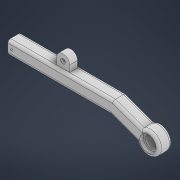
# Autodesk Inventor part: Fahrwerk_rocker_hinten
Saved by Autodesk Inventor 2021 (Build 250183000, 183)
## iProperties
Created: 2020-12-28
Part Number: Fahrwerk_rocker_hinten
Material: Generisch
Document SubType Name: Modeling
Designer: laure
Density: 1 g/cm^3
Appearance: Vorgabe
Author: laure
Autodesk Inventor part; units mm, degrees
ref_plane "YZ Plane" through (0, 0, 0) normal (1, 0, 0) x (0, 1, 0)
ref_plane "XZ Plane" through (0, 0, 0) normal (0, 1, 0) x (-1, 0, 0)
ref_plane "XY Plane" through (0, 0, 0) normal (0, 0, 1) x (1, 0, 0)
sketch "Skizze1" plane through (0, 0, 0) normal (0, 0, 1) x (1, 0, 0)
  line L0 (-110, 10) -> (50, 10)
  line L1 (46.4735, -10) -> (-110, -10)
  line L2 (-153.2763, 0) -> (149.6579, 0) projected
  line L3 (99.5412, -29.3151) -> (46.4735, -10)
  line L4 (50, 10) -> (106.3816, -10.5212)
  line L5 (106.3816, -10.5212) -> (99.5412, -29.3151)
  line L6 (0, -40.3885) -> (0, 37.1255) projected
  line L7 (-110, 10) -> (-110, -10)
  point P0 (0, 0)
  dimension "d5" = 20
  dimension "d56" = 0
  dimension "d57" = 0
  dimension "d58" = 60
  dimension "d138" = 160
  dimension "d140" = 20
  dimension "d141" = 10
  dimension "d142" = 110
  dimension "d143" = 50
  dimension "d144" = 10
  constraints: 12 end point, 2 parallel, 2 perpendicular, 1 horizontal, 1 other
  measures "d5" distance between parallel lines of L4 L3
  measures "d56" distance from line of L0 L4.start
  measures "d57" distance of L0.end L4.start
  measures "d58" distance from line of L4.start L5
  measures "d138" distance from line of L7 L0.end
  measures "d140" angle of L6 L5
  measures "d141" distance between parallel lines of L2 L0
  measures "d142" distance between parallel lines of L6 L7
  measures "d143" distance from line of point (50, 10) L6
  measures "d144" distance from line of point (50, 10) L2
sketch "Skizze4" plane through (0, 0, 0) normal (0, 0, 1) x (1, 0, 0)
  line L0 (-40, 10) -> (-20, 10)
  line L1 (-20, 10) -> (-20, 20)
  line L2 (-30, 30) -> (-30, 30)
  line L3 (-40, 20) -> (-40, 10)
  arc A0 (-30, 30) -> (-40, 20) centre (-30, 20) ccw
  arc A1 (-20, 20) -> (-30, 30) centre (-30, 20) ccw
  line L4 (-50.4853, 0) -> (8.4142, 0) projected
  line L5 (0, -6.4142) -> (0, 38.4853) projected
  line L6 (-35, 25) -> (-25, 25)
  line L7 (-25, 25) -> (-25, 15)
  line L8 (-25, 15) -> (-35, 15)
  line L9 (-35, 15) -> (-35, 25)
  line L10 (-35, 25) -> (-25, 15) construction
  line L11 (-25, 25) -> (-35, 15) construction
  point P0 (0, 0)
  point P1 (-30, 30)
  dimension "d74" = 20
  dimension "d75" = 20
  dimension "d78" = 10
  dimension "d116" = 10
  dimension "d160" = 10
  dimension "d161" = 10
  dimension "d162" = 20
  dimension "d167" = 10
  constraints: 20 end point, 4 parallel, 4 point on circle, 4 tangent, 2 centre point, 2 horizontal, 2 midpoint, 2 perpendicular, 1 concentric
  measures "d74" distance between parallel lines of L1 L3
  measures "d75" distance between parallel lines of L0 L2
  measures "d78" radius of A0
  measures "d116" distance between parallel lines of L0 L4
  measures "d160" distance of L7.end L8.end
  measures "d161" distance of L6.end L7.end
  measures "d162" distance between parallel lines of L5 L1
  measures "d167" distance from line of L0 A1.centre
extrude "Extrusion1" add sketch "Skizze1" against normal mid plane 20
sketch "Skizze13" plane through (0, 0, -10) normal (0, 0, -1) x (-1, 0, 0)
  line L0 (-106.3816, -10.5212) -> (-99.5412, -29.3151) projected
  circle A0 centre (-102.9614, -19.9181) radius 12.15
  circle A1 centre (-102.9614, -19.9181) radius 17
  point P0 (0, 0)
  point P1 (-105.5778, -12.7295)
  point P2 (-100.3449, -27.1068)
  dimension "d148" = 24.3
  dimension "d149" = 34
  constraints: 2 centre point, 1 coincident, 1 midpoint
  measures "d148" diameter of A0
  measures "d149" diameter of A1
extrude "Extrusion13" add sketch "Skizze13" against normal blind 20
extrude "Extrusion14" cut sketch "Skizze13" against normal up to surface (20 mm away) contours A0
shell "Wandung2" thickness 2.6 removed faces 1 at (-110, -3.3333, -3.3333)
extrude "Extrusion11" add sketch "Skizze4" against normal mid plane 12 contours L3 A0 A1 L1 L0 | L6 L7 L8 L9
sketch "Skizze12" plane through (0, 0, 10) normal (0, 0, 1) x (1, 0, 0)
  circle A0 centre (-104, 0) radius 1.6
  line L0 (-110, 6) -> (49.2947, 6) projected
  line L1 (-110, 10) -> (-110, -10) projected
  line L2 (50, 10) -> (-110, 10) projected
  point P0 (0, 0)
  point P1 (-110, -6)
  dimension "d133" = 3.2
  dimension "d135" = 6
  dimension "d147" = 10
  constraints: 1 centre point
  measures "d133" diameter of A0
  measures "d135" distance from line of L1 A0.centre
  measures "d147" distance from line of A0.centre L2
extrude "Extrusion12" cut sketch "Skizze12" against normal up to surface (20 mm away)
sketch "Skizze14" plane through (0, 0, 0) normal (0, 0, 1) x (1, 0, 0)
  circle A0 centre (102.9614, -19.9181) radius 12.15 projected
  circle A1 centre (102.9614, -19.9181) radius 9
  point P0 (0, 0)
  dimension "d157" = 18
  constraints: 1 centre point, 1 coincident
  measures "d157" diameter of A1
extrude "Extrusion15" add sketch "Skizze14" along normal mid plane 10
extrude "Extrusion16" cut sketch "Skizze4" against normal blind 6 contours L6 L7 L8 L9
sketch "Skizze15" plane through (0, 0, 6) normal (0, 0, 1) x (1, 0, 0)
  circle A0 centre (-30, 20) radius 3.5
  line L0 (-20, 10) -> (-20, 20) projected
  line L1 (-20, 10) -> (-40, 10) projected
  point P0 (0, 0)
  dimension "d165" = 7
  dimension "d166" = 10
  dimension "d168" = 10
  constraints: 1 centre point
  measures "d165" diameter of A0
  measures "d166" distance from line of L0 A0.centre
  measures "d168" distance from line of L1 A0.centre
extrude "Extrusion17" cut sketch "Skizze15" against normal blind 3
sketch "Skizze16" plane through (-30, 20, 3) normal (0, 0, 1) x (1, 0, 0)
  circle A0 centre (0, 0) radius 1.6
  line L0 (10, -10) -> (10, 0) projected
  line L1 (10, -10) -> (-10, -10) projected
  point P0 (30, -20)
  dimension "d171" = 3.2
  dimension "d172" = 10
  dimension "d173" = 10
  constraints: 1 centre point
  measures "d171" diameter of A0
  measures "d172" distance from line of L0 A0.centre
  measures "d173" distance from line of L1 A0.centre
extrude "Extrusion18" cut sketch "Skizze16" against normal blind 3
fillet "Rundung7" radius 4 10 edges at (71.7315, 2.0904, -10) (71.7315, 2.0904, 10) (-30, 10, 10) (-30, 10, -10) (-31.7633, -10, -10) (66.548, -17.3065, -10) (-31.7633, -10, 10) (66.548, -17.3065, 10) (118.9361, -25.7325, 10) (118.9361, -25.7325, -10)
